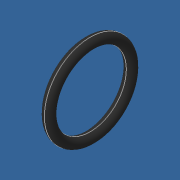
# Autodesk Inventor part: O-Ring
Saved by Autodesk Inventor 2018 (Build 220112000, 112)
## iProperties
Created: 2018-11-04
Part Number: O-Ring
Material: Gummi, Silikon
Document SubType Name: Modeling
Designer: M.Knabel
Density: 1.25 g/cm^3
Appearance: Gummi - schwarz
Author: M.Knabel
Autodesk Inventor part; units mm, degrees
ref_plane "YZ Plane" through (0, 0, 0) normal (1, 0, 0) x (0, 1, 0)
ref_plane "XZ Plane" through (0, 0, 0) normal (0, 1, 0) x (-1, 0, 0)
ref_plane "XY Plane" through (0, 0, 0) normal (0, 0, 1) x (1, 0, 0)
sketch "Skizze1" plane through (0, 0, 0) normal (0, 0, 1) x (1, 0, 0)
  line L0 (-1.7521, 0) -> (1.7479, 0) projected
  line L1 (0, -2.1617) -> (0, 12.97) projected
  arc A0 (0, 10.8042) -> (0, 8.5042) centre (-0.0979, 9.6542) ccw
  line L2 (0, 10.8042) -> (0.0979, 10.8042)
  line L3 (0, 8.5042) -> (0.0979, 8.5042)
  arc A1 (0.0979, 8.5042) -> (0.0979, 10.8042) centre (0.0979, 9.6542) ccw
  point P0 (0, 0)
  dimension "d2" = 17
  dimension "d4" = 2.3
  dimension "d5" = 2.5
  constraints: 4 end point, 4 point on circle, 2 centre point, 2 horizontal, 2 point on line, 2 tangent, 1 symmetric about line
  measures "d4" distance between parallel lines of L2 L3
revolve "Umdrehung2" add sketch "Skizze1" angle 360 about axis through (-10, 0, 0) along (1, 0, 0)
